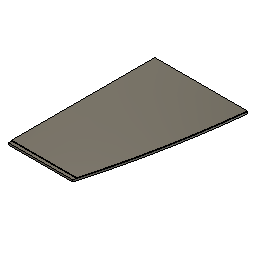
oceaan-25-floor_1 v2 (Autodesk Fusion 360 design; units mm, degrees)
Autodesk Fusion 360 part; units mm, degrees
note: some values were not read from the file. Set by a fixed rule: which sketch regions a step uses.
sketch "Sketch1" plane through (0, 0, 0) normal (0, 1, 0) x (1, 0, 0)
  line L0 (30, -14) -> (30, 656)
  line L1 (30, 656) -> (454, 656)
  line L2 (30, 0) -> (327, 0)
  line L3 (30, -14) -> (324, -14)
  arc A0 (324, -14) -> (454, 656) centre (-3623.5497, 1099.5544) ccw
  dimension "d1" = 670
  dimension "d2" = 656
  dimension "d4" = 424
  dimension "d6" = 297
  dimension "d7" = 294
  constraint vertical L0
  constraint perpendicular L0 L2
  constraint perpendicular L0 L3
  constraint perpendicular L0 L1
  measures "d1" distance of L0.start L0.end
  measures "d2" distance of L2.start L0.end
  measures "d4" distance of L0.end L1.end
  measures "d6" distance of L2.start L2.end
  measures "d7" distance of L0.start L3.end
sketch "Sketch2" plane through (0, 0, 0) normal (0, 1, 0) x (-1, 0, 0)
  arc A0 (-324, 14) -> (-454, -656) centre (3623.5497, -1099.5544) ccw
  line L0 (-30, 0) -> (-327, 0)
  line L1 (-30, 14) -> (-30, -656)
  line L2 (-327.9225, 0) -> (-30, 0)
  line L3 (-30, 0) -> (-30, -656)
  line L4 (-30, -656) -> (-454, -656)
  arc A1 (-327.9225, 0) -> (-454, -656) centre (3624.5853, -1099.7535) ccw
  point P0 (-30, 0)
  constraint coincident A0 L2.start
  constraint coincident L0 L2.start
  constraint coincident P0 L0.start
  constraint coincident L1.end L3.end
  constraint coincident A0.end L4.end
extrude "Extrude1" add sketch "Sketch1" sketch "Sketch2" against normal blind 9 of sketch 2
extrude "Extrude2" add sketch "Sketch2" along normal blind 3.5
equation "d2 = 644 mm + 12 mm"
